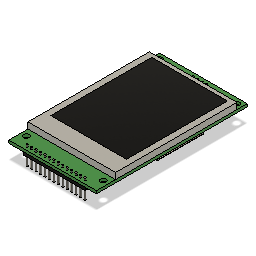
_2,8Zoll TFT SPI.7f793562-e44e-44ae-986e-20ae59d8bd2c (Autodesk Fusion 360 design; units mm, degrees)
Autodesk Fusion 360 part; units mm, degrees
sketch "Skizze1" plane through (0, 0, 0) normal (0, 1, 0) x (1, 0, 0)
  line L0 (0, 0) -> (50, 0)
  line L1 (50, 0) -> (50, 86)
  line L2 (50, 86) -> (0, 86)
  line L3 (0, 86) -> (0, 0)
  circle A0 centre (3, 83) radius 1.6
  circle A1 centre (47, 83) radius 1.6
  circle A2 centre (47, 6.92) radius 1.6
  circle A3 centre (3, 6.92) radius 1.6
  circle A4 centre (8.49, 2) radius 0.5
  circle A5 centre (11.03, 2) radius 0.5
  circle A6 centre (13.57, 2) radius 0.5
  circle A7 centre (16.11, 2) radius 0.5
  circle A8 centre (18.65, 2) radius 0.5
  circle A9 centre (21.19, 2) radius 0.5
  circle A10 centre (23.73, 2) radius 0.5
  circle A11 centre (26.27, 2) radius 0.5
  circle A12 centre (28.81, 2) radius 0.5
  circle A13 centre (31.35, 2) radius 0.5
  circle A14 centre (33.89, 2) radius 0.5
  circle A15 centre (36.43, 2) radius 0.5
  circle A16 centre (38.97, 2) radius 0.5
  circle A17 centre (41.51, 2) radius 0.5
  line L4 (25, 86) -> (25, 0) construction
  line L5 (0, 84) -> (50, 84) construction
  circle A18 centre (23.73, 84) radius 0.5
  circle A19 centre (26.27, 84) radius 0.5
  circle A20 centre (28.81, 84) radius 0.5
  circle A21 centre (21.19, 84) radius 0.5
  dimension "d1" = 50
  dimension "d2" = 86
  dimension "d3" = 3.2
  dimension "d4" = 3.2
  dimension "d5" = 3.2
  dimension "d6" = 3.2
  dimension "d7" = 6.92
  dimension "d8" = 6.92
  dimension "d9" = 3
  dimension "d10" = 3
  dimension "d11" = 3
  dimension "d12" = 3
  dimension "d13" = 3
  dimension "d14" = 3
  dimension "d15" = 1
  dimension "d16" = 8.49
  dimension "d17" = 2
  dimension "d20" = 2.54
  dimension "d21" = 0
  dimension "d22" = 8.49
  dimension "d36" = 2
  dimension "d37" = 1
  dimension "d38" = 1
  dimension "d39" = 1
  dimension "d40" = 1
  dimension "d41" = 1.27
  dimension "d42" = 1.27
  dimension "d43" = 2.54
  dimension "d44" = 2.54
  measures "d3" diameter of A0
  measures "d4" diameter of A1
  measures "d5" diameter of A2
  measures "d6" diameter of A3
  measures "d15" diameter of A4
  measures "d36" distance of L2 L5
  measures "d37" diameter of A18
  measures "d38" diameter of A19
  measures "d39" diameter of A20
  measures "d40" diameter of A21
extrude "Extrusion1" add sketch "Skizze1" along normal blind 1.6 makes body 1
sketch "Skizze2" plane through (0, 1.6, 0) normal (0, 1, 0) x (-1, 0, 0)
  circle A0 centre (-16.11, -2) radius 0.5
  circle A1 centre (-18.65, -2) radius 0.5
  circle A2 centre (-21.19, -2) radius 0.5
  circle A3 centre (-23.73, -2) radius 0.5
  circle A4 centre (-26.27, -2) radius 0.5
  circle A5 centre (-13.57, -2) radius 0.5
  circle A6 centre (-11.03, -2) radius 0.5
  circle A7 centre (-8.49, -2) radius 0.5
  circle A8 centre (-3, -6.92) radius 1.6
  circle A9 centre (-47, -6.92) radius 1.6
  circle A10 centre (-47, -83) radius 1.6
  circle A11 centre (-3, -83) radius 1.6
  circle A12 centre (-28.81, -2) radius 0.5
  circle A13 centre (-33.89, -2) radius 0.5
  circle A14 centre (-36.43, -2) radius 0.5
  circle A15 centre (-38.97, -2) radius 0.5
  circle A16 centre (-41.51, -2) radius 0.5
  circle A17 centre (-31.35, -2) radius 0.5
  line L0 (0, -86) -> (0, 0)
  line L1 (0, 0) -> (-50, 0)
  line L2 (-50, 0) -> (-50, -86)
  line L3 (-50, -86) -> (0, -86)
  line L4 (0, -80.2) -> (-50, -80.2)
  line L5 (-50, -80.2) -> (-50, -10.9)
  line L6 (-50, -10.9) -> (0, -10.9)
  line L7 (0, -10.9) -> (0, -80.2)
  circle A18 centre (-28.81, -84) radius 0.5
  circle A19 centre (-23.73, -84) radius 0.5
  circle A20 centre (-26.27, -84) radius 0.5
  circle A21 centre (-21.19, -84) radius 0.5
  dimension "d25" = 5.8
  dimension "d26" = 10.9
  measures "d25" distance of L3 L4
  measures "d26" distance of L1 L6
extrude "Extrusion2" add sketch "Skizze2" along normal blind 3.54 separate body contours L0 L2 L4 L5 L6 L7 makes body 2
sketch "Skizze3" plane through (0, 5.14, 0) normal (0, 1, 0) x (-1, 0, 0)
  line L0 (0, -10.9) -> (-50, -10.9)
  line L1 (-50, -10.9) -> (-50, -80.2)
  line L2 (-50, -80.2) -> (0, -80.2)
  line L3 (0, -80.2) -> (0, -10.9)
  line L4 (-3.4, -78.15) -> (-46.6, -78.15)
  line L5 (-46.6, -78.15) -> (-46.6, -20.55)
  line L6 (-46.6, -20.55) -> (-3.4, -20.55)
  line L7 (-3.4, -20.55) -> (-3.4, -78.15)
  line L8 (-25, -80.2) -> (-25, -10.9) construction
  dimension "d29" = 43.2
  dimension "d30" = 57.6
  dimension "d31" = 21.6
  dimension "d32" = 2.05
  dimension "d33" = 3.4
  measures "d29" distance of origin
  measures "d30" distance of L4 L6
  measures "d31" distance of L7 L8
  measures "d32" distance of L2 L4
  measures "d33" distance of L1 L5
extrude "Extrusion3" cut sketch "Skizze3" against normal blind 0.01 contours L4 L5 L6 L7 bodies 2
sketch "Skizze4" plane through (0, 0, 0) normal (0, -1, 0) x (1, 0, 0)
  circle A0 centre (28.81, -84) radius 0.5
  circle A1 centre (41.51, -2) radius 0.5
  circle A2 centre (23.73, -84) radius 0.5
  circle A3 centre (26.27, -84) radius 0.5
  circle A4 centre (23.73, -2) radius 0.5
  circle A5 centre (21.19, -84) radius 0.5
  circle A6 centre (26.27, -2) radius 0.5
  circle A7 centre (28.81, -2) radius 0.5
  circle A8 centre (31.35, -2) radius 0.5
  circle A9 centre (33.89, -2) radius 0.5
  circle A10 centre (36.43, -2) radius 0.5
  circle A11 centre (38.97, -2) radius 0.5
  circle A12 centre (21.19, -2) radius 0.5
  circle A13 centre (18.65, -2) radius 0.5
  circle A14 centre (16.11, -2) radius 0.5
  circle A15 centre (13.57, -2) radius 0.5
  circle A16 centre (11.03, -2) radius 0.5
  circle A17 centre (8.49, -2) radius 0.5
  circle A18 centre (3, -6.92) radius 1.6
  circle A19 centre (47, -6.92) radius 1.6
  circle A20 centre (47, -83) radius 1.6
  circle A21 centre (3, -83) radius 1.6
  line L0 (0, 0) -> (0, -86)
  line L1 (0, -86) -> (50, -86)
  line L2 (50, -86) -> (50, 0)
  line L3 (50, 0) -> (0, 0)
  line L4 (31.4, -36.8) -> (48, -36.8)
  line L5 (48, -36.8) -> (48, -63.3)
  line L6 (48, -63.3) -> (31.4, -63.3)
  line L7 (31.4, -63.3) -> (31.4, -36.8)
  dimension "d45" = 16.6
  dimension "d46" = 2
  dimension "d47" = 36.8
  dimension "d48" = 22.7
  measures "d45" distance of L5 L7
  measures "d46" distance of L2 L5
  measures "d47" distance of L3 L4
  measures "d48" distance of L1 L6
extrude "Extrusion4" add sketch "Skizze4" along normal blind 2.95 separate body contours L4 L5 L6 L7 makes body 3
sketch "Skizze5" plane through (48, 0, 0) normal (1, 0, 0) x (0, 0, -1)
  line L0 (63.3, 0) -> (36.8, 0)
  line L1 (36.8, 0) -> (36.8, -2.95)
  line L2 (36.8, -2.95) -> (63.3, -2.95)
  line L3 (63.3, -2.95) -> (63.3, 0)
  line L4 (38, -0.25) -> (62.1, -0.25)
  line L5 (62.1, -0.25) -> (62.1, -2.75)
  line L6 (62.1, -2.75) -> (38, -2.75)
  line L7 (38, -2.75) -> (38, -0.25)
  dimension "d51" = 0.2
  dimension "d52" = 1.2
  dimension "d53" = 1.2
  dimension "d54" = 2.5
  measures "d51" distance of L2 L6
  measures "d52" distance of L3 L5
  measures "d53" distance of L1 L7
  measures "d54" distance of L4 L6
extrude "Extrusion5" cut sketch "Skizze5" against normal blind 15 contours L4 L5 L6 L7 bodies 3
sketch "Skizze6" plane through (0, 0, 0) normal (0, -1, 0) x (1, 0, 0)
  circle A0 centre (28.81, -84) radius 0.5
  circle A1 centre (41.51, -2) radius 0.5
  circle A2 centre (23.73, -84) radius 0.5
  circle A3 centre (26.27, -84) radius 0.5
  circle A4 centre (23.73, -2) radius 0.5
  circle A5 centre (21.19, -84) radius 0.5
  circle A6 centre (26.27, -2) radius 0.5
  circle A7 centre (28.81, -2) radius 0.5
  circle A8 centre (31.35, -2) radius 0.5
  circle A9 centre (33.89, -2) radius 0.5
  circle A10 centre (36.43, -2) radius 0.5
  circle A11 centre (38.97, -2) radius 0.5
  circle A12 centre (21.19, -2) radius 0.5
  circle A13 centre (18.65, -2) radius 0.5
  circle A14 centre (16.11, -2) radius 0.5
  circle A15 centre (13.57, -2) radius 0.5
  circle A16 centre (11.03, -2) radius 0.5
  circle A17 centre (8.49, -2) radius 0.5
  circle A18 centre (3, -6.92) radius 1.6
  circle A19 centre (47, -6.92) radius 1.6
  circle A20 centre (47, -83) radius 1.6
  circle A21 centre (3, -83) radius 1.6
  line L0 (0, 0) -> (0, -86)
  line L1 (0, -86) -> (50, -86)
  line L2 (50, -86) -> (50, 0)
  line L3 (50, 0) -> (0, 0)
  circle A22 centre (8.49, -2) radius 0.5
  circle A23 centre (11.03, -2) radius 0.5
  circle A24 centre (13.57, -2) radius 0.5
  circle A25 centre (16.11, -2) radius 0.5
  circle A26 centre (18.65, -2) radius 0.5
  circle A27 centre (21.19, -2) radius 0.5
  circle A28 centre (23.73, -2) radius 0.5
  circle A29 centre (26.27, -2) radius 0.5
  circle A30 centre (28.81, -2) radius 0.5
  circle A31 centre (31.35, -2) radius 0.5
  circle A32 centre (33.89, -2) radius 0.5
  circle A33 centre (36.43, -2) radius 0.5
  circle A34 centre (38.97, -2) radius 0.5
  circle A35 centre (41.51, -2) radius 0.5
extrude "Extrusion6" add sketch "Skizze6" along normal blind 8 and the other way blind 2.8 separate body contours A1 A35 | A4 A28 | A6 A29 | A7 A30 | A8 A31 | A9 A32 | A10 A33 | A11 A34 | A12 A27 | A13 A26 | A14 A25 | A15 A24 | A16 A23 | A17 A22 makes body 4 at (36.0809, -5.3333, -1.6421) makes body 5 at (26.4054, -5.3333, -1.5187) makes body 6 at (16.4408, -2.6667, -2.3749) makes body 7 at (8.9894, -5.3333, -2.0249) makes body 8 at (18.3009, -5.3333, -1.6421) makes body 9 at (28.9454, -5.3333, -1.5187) makes body 10 at (38.6209, -5.3333, -1.6421) makes body 11 at (33.5409, -5.3333, -1.6421) makes body 12 at (23.8654, -5.3333, -1.5187) makes body 13 at (14.0694, -5.3333, -2.0249) makes body 14 at (11.5294, -5.3333, -2.0249) makes body 15 at (21.3254, -5.3333, -1.5187) makes body 16 at (31.8494, -5.3333, -2.0249) makes body 17 at (41.1609, -5.3333, -1.6421)
sketch "Skizze7" plane through (0, 0, 0) normal (0, -1, 0) x (1, 0, 0)
  circle A0 centre (28.81, -84) radius 0.5
  circle A1 centre (41.51, -2) radius 0.5
  circle A2 centre (23.73, -84) radius 0.5
  circle A3 centre (26.27, -84) radius 0.5
  circle A4 centre (23.73, -2) radius 0.5
  circle A5 centre (21.19, -84) radius 0.5
  circle A6 centre (26.27, -2) radius 0.5
  circle A7 centre (28.81, -2) radius 0.5
  circle A8 centre (31.35, -2) radius 0.5
  circle A9 centre (33.89, -2) radius 0.5
  circle A10 centre (36.43, -2) radius 0.5
  circle A11 centre (38.97, -2) radius 0.5
  circle A12 centre (21.19, -2) radius 0.5
  circle A13 centre (18.65, -2) radius 0.5
  circle A14 centre (16.11, -2) radius 0.5
  circle A15 centre (13.57, -2) radius 0.5
  circle A16 centre (11.03, -2) radius 0.5
  circle A17 centre (8.49, -2) radius 0.5
  circle A18 centre (3, -6.92) radius 1.6
  circle A19 centre (47, -6.92) radius 1.6
  circle A20 centre (47, -83) radius 1.6
  circle A21 centre (3, -83) radius 1.6
  line L0 (0, 0) -> (0, -86)
  line L1 (0, -86) -> (50, -86)
  line L2 (50, -86) -> (50, 0)
  line L3 (50, 0) -> (0, 0)
  line L4 (7.29, -0.8) -> (42.71, -0.8)
  line L5 (42.71, -0.8) -> (42.71, -3.2)
  line L6 (42.71, -3.2) -> (7.29, -3.2)
  line L7 (7.29, -3.2) -> (7.29, -0.8)
  dimension "d59" = 1.2
  dimension "d60" = 1.2
  dimension "d61" = 1.2
  dimension "d62" = 1.2
  measures "d59" distance of L4
  measures "d60" distance of L6
  measures "d61" distance of L7
  measures "d62" distance of L5
extrude "Extrusion7" add sketch "Skizze7" along normal blind 2.4 separate body contours L4 L5 L6 L7 makes body 18
equation "d31 = ( 43.2 / 2 ) * 1 mm"
